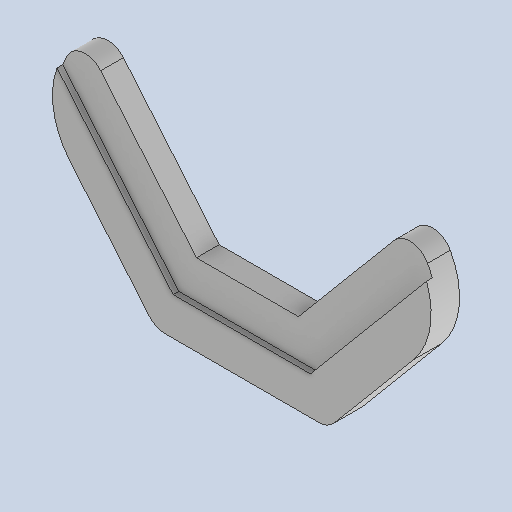
# Autodesk Inventor part: ДМФ 033 держатель лотка v2.0
Saved by Autodesk Inventor 2025 (Build 290162010, 162A)
## iProperties
Created: 2024-05-13
Part Number: ДМФ 033 держатель лотка v2.0
Material: Generic
Document SubType Name: Sheet Metal
Designer: admin
Density: 1 g/cm^3
Appearance: Default
Stock Number: ДМФ 033 держатель лотка
Flat Pattern Width: 17.1308 cm
Flat Pattern Length: 16.5929 cm
Flat Pattern Area: 284.248 cm^2
Sheet Metal Rule: Default
Sheet Metal Width: 171,308 mm
Sheet Metal Length: 165,929 mm
Sheet Metal Area: 28424,842 mm^2
Author: admin
Autodesk Inventor part; units mm, degrees
ref_plane "YZ Plane" through (0, 0, 0) normal (1, 0, 0) x (0, 1, 0)
ref_plane "XZ Plane" through (0, 0, 0) normal (0, 1, 0) x (-1, 0, 0)
ref_plane "XY Plane" through (0, 0, 0) normal (0, 0, 1) x (1, 0, 0)
sketch "Sketch1" plane through (0, 0, 0) normal (0, 1, 0) x (-1, 0, 0)
  line L0 (-26.95, 0) -> (26.95, 0)
  line L1 (-26.95, 0) -> (-85.687, 70)
  line L2 (85.687, 70) -> (26.95, 0)
  line L3 (90.6172, 13.6467) -> (45.6023, -40)
  line L4 (45.6023, -40) -> (-45.6023, -40)
  line L5 (-45.6023, -40) -> (-90.6172, 13.6467)
  line L6 (0, 0) -> (0, -40) construction
  arc A0 (90.6172, 13.6467) -> (85.687, 70) centre (59.9755, 39.3582) ccw
  arc A1 (-85.687, 70) -> (-90.6172, 13.6467) centre (-59.9755, 39.3582) ccw
  point P0 (0, 70)
  dimension "d1" = 53.9
  dimension "d3" = 40
  dimension "d5" = 40
  dimension "d16" = 130
  dimension "d17" = 70
  constraints: 14 end point, 4 point on circle, 2 centre point, 2 line through centre, 2 midpoint, 2 parallel, 2 tangent, 2 vertical alignment, 1 coincident, 1 equal length, 1 horizontal, 1 perpendicular, 1 other
  measures "d1" distance of L0.start L0.end
  measures "d3" distance between parallel lines of L4 L0
  measures "d5" distance between parallel lines of L3 L2
  measures "d16" angle of L0 L2
  measures "d17" distance from line of L0 L2.start
extrude "Extrusion1" add sketch "Sketch1" along normal blind 15
sketch "Sketch2" plane through (0, 0, 0) normal (0, -1, 0) x (1, 0, 0)
  line L0 (-26.95, 0) -> (26.95, 0) projected
  line L1 (-85.687, 70) -> (-26.95, 0) projected
  line L2 (-45.6023, -40) -> (-90.6172, 13.6467) construction
  line L3 (45.6023, -40) -> (-45.6023, -40) construction
  line L4 (90.6172, 13.6467) -> (45.6023, -40) construction
  line L5 (26.95, 0) -> (85.687, 70) projected
  line L6 (-97.5632, 53.039) -> (-36.2762, -20)
  line L7 (-36.2762, -20) -> (36.2762, -20)
  line L8 (36.2762, -20) -> (97.5632, 53.039)
  line L9 (-85.687, 70) -> (-26.95, 0) projected
  line L10 (26.95, 0) -> (85.687, 70) projected
  arc A0 (-85.687, 70) -> (-90.6172, 13.6467) centre (-59.9755, 39.3582) ccw projected
  arc A1 (90.6172, 13.6467) -> (85.687, 70) centre (59.9755, 39.3582) ccw projected
  point P0 (0, 0)
  dimension "d8" = 20
  dimension "d9" = 20
  dimension "d10" = 20
  constraints: 6 end point, 2 parallel, 2 point on circle, 1 horizontal
  measures "d8" distance between parallel lines of L7 L0
  measures "d9" distance between parallel lines of L1 L6
  measures "d10" distance between parallel lines of L5 L8
extrude "Extrusion2" cut sketch "Sketch2" against normal blind 3
fillet "Fillet1" radius 10.7 4 edges at (-85.687, 9, 70) (85.687, 9, 70) (-45.6023, 7.5, -40) (45.6023, 7.5, -40)
equation "\"d5\" = d3"
equation "\"d16\" = Лоток_угол"
equation "\"d9\" = d8"
equation "\"d10\" = d8"
equation "\"BendRadius\" = Thickness"
equation "\"BendReliefWidth\" = Thickness"
equation "\"BendReliefDepth\" = 0.5 * Thickness"
equation "\"TransitionRadius\" = BendRadius"
equation "\"JacobiRadiusSize\" = BendRadius"
equation "\"GapSize\" = Thickness"
equation "\"Лоток_угол\" = 130deg"
equation "\"Thickness\" = 15"
body "Solid1"
